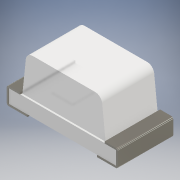
# Autodesk Inventor part: 63-0001
Saved by Autodesk Inventor 2018 (Build 220112000, 112)
## iProperties
Created: 2019-09-26
Part Number: 63-0001
Material: ABS Plastic
Document SubType Name: Modeling
Designer: Bradley
Density: 1.06 g/cm^3
Appearance: Smooth - White
Author: Bradley
Autodesk Inventor part; units mm, degrees
ref_plane "YZ Plane" through (0, 0, 0) normal (1, 0, 0) x (0, 1, 0)
ref_plane "XZ Plane" through (0, 0, 0) normal (0, 1, 0) x (-1, 0, 0)
ref_plane "XY Plane" through (0, 0, 0) normal (0, 0, 1) x (1, 0, 0)
sketch "Sketch1" plane through (0, 0, 0) normal (0, 0, 1) x (1, 0, 0)
  line L0 (-0.775, -0.395) -> (0.775, -0.395)
  line L1 (0.775, -0.395) -> (0.775, 0.395)
  line L2 (0.775, 0.395) -> (-0.775, 0.395)
  line L3 (-0.775, 0.395) -> (-0.775, -0.395)
  line L4 (-0.775, -0.395) -> (0.775, 0.395) construction
  line L5 (0.775, -0.395) -> (-0.775, 0.395) construction
  point P0 (0, 0)
  dimension "d0" = 1.55
  dimension "d1" = 0.79
  constraints: 12 end point, 2 midpoint, 2 parallel, 1 horizontal, 1 perpendicular
  measures "d0" distance of L2.end L1.end
  measures "d1" distance of L1.end L0.end
extrude "Extrusion1" add sketch "Sketch1" along normal blind 0.2
sketch "Sketch2" plane through (0, 0, 0) normal (0, 1, 0) x (-1, 0, 0)
  line L0 (0.775, 0) -> (-0.775, 0) projected
  line L1 (-0.775, 0) -> (-0.775, 0.2) projected
  line L2 (0.775, 0.2) -> (-0.775, 0.2) projected
  line L3 (0.775, 0) -> (0.775, 0.2) projected
  line L4 (0.6, 0.2) -> (0.55, 0.6608)
  arc A0 (0.55, 0.6608) -> (0.4506, 0.75) centre (0.4506, 0.65) ccw
  line L5 (0.4506, 0.75) -> (-0.4506, 0.75)
  arc A1 (-0.4506, 0.75) -> (-0.55, 0.6608) centre (-0.4506, 0.65) ccw
  line L6 (-0.55, 0.6608) -> (-0.6, 0.2)
  line L7 (0.5995, 0.205) -> (-0.5995, 0.205)
  point P0 (0, 0)
  point P1 (0, 0.75)
  point P2 (0, 0.2)
  dimension "d7" = 1.2
  dimension "d8" = 1.1
  dimension "d9" = 0.1
  dimension "d22" = 0.75
  dimension "d23" = 0.005
  constraints: 8 end point, 4 point on circle, 4 point on line, 4 tangent, 2 centre point, 2 horizontal, 2 midpoint, 1 equal length, 1 equal radius, 1 vertical alignment
  measures "d7" distance of L6.end L4.start
  measures "d8" distance of L6.start L4.end
  measures "d9" radius of A0
  measures "d22" distance between parallel lines of L0 L5
  measures "d23" distance between parallel lines of L2 L7
extrude "Extrusion3" add sketch "Sketch2" along normal mid plane 0.75 contours L7 L6 A1 L5 A0 L4
sketch "Sketch3" plane through (-0.775, 0, 0) normal (0, -1, 0) x (1, 0, 0)
  line L0 (0, 0) -> (1.55, 0) projected
  line L1 (1.55, 0) -> (1.55, 0.2) projected
  line L2 (0, 0.2) -> (1.55, 0.2) projected
  line L3 (0, 0) -> (0, 0.2) projected
  line L4 (0, 0.2) -> (1.55, 0.2) projected
  line L5 (0.165, 0.2) -> (0.165, 0.225)
  line L6 (0.165, 0.225) -> (0, 0.225)
  arc A0 (0, 0.225) -> (-0.025, 0.2) centre (0, 0.2) ccw
  line L7 (-0.025, 0.2) -> (-0.025, 0)
  arc A1 (-0.025, 0) -> (0, -0.025) centre (0, 0) ccw
  line L8 (0, -0.025) -> (0.275, -0.025)
  line L9 (0.275, -0.025) -> (0.275, 0)
  line L10 (0, 0) -> (1.55, 0) projected
  line L11 (1.275, 0) -> (1.275, -0.025)
  line L12 (1.275, -0.025) -> (1.55, -0.025)
  arc A2 (1.55, -0.025) -> (1.575, 0) centre (1.55, 0) ccw
  line L13 (1.575, 0) -> (1.575, 0.2)
  arc A3 (1.575, 0.2) -> (1.55, 0.225) centre (1.55, 0.2) ccw
  line L14 (1.55, 0.225) -> (1.385, 0.225)
  line L15 (1.385, 0.225) -> (1.385, 0.2)
  point P0 (0.775, 0)
  dimension "d13" = 1.6
  dimension "d14" = 0.3
  dimension "d15" = 0.19
  constraints: 20 end point, 8 point on circle, 8 point on line, 7 perpendicular, 7 tangent, 4 centre point, 4 coincident, 2 collinear, 1 vertical
  measures "d13" distance between parallel lines of L13 L7
  measures "d14" distance between parallel lines of L7 L9
  measures "d15" distance between parallel lines of L7 L5
extrude "Extrusion4" add sketch "Sketch3" along normal mid plane 0.8 contours L0 L9 L8 A1 L7 A0 L6 L5 L2 L3 | L0 L1 L2 L15 L14 A3 L13 A2 L12 L11
sketch "Sketch4" plane through (0, 0, 0.2) normal (0, 0, 1) x (1, 0, 0)
  line L0 (-0.775, 0.4) -> (-0.775, -0.4) projected
  line L1 (-0.61, -0.4) -> (-0.775, -0.4) projected
  line L2 (-0.61, 0.4) -> (-0.61, -0.4) projected
  line L3 (-0.775, 0.4) -> (-0.61, 0.4) projected
  line L4 (0.61, 0.4) -> (0.61, -0.4) projected
  line L5 (0.775, -0.4) -> (0.61, -0.4) projected
  line L6 (0.775, 0.4) -> (0.775, -0.4) projected
  line L7 (0.61, 0.4) -> (0.775, 0.4) projected
  line L8 (-0.4, -0.15) -> (-0.1, -0.15)
  line L9 (-0.1, -0.15) -> (-0.1, 0.15)
  line L10 (-0.1, 0.15) -> (-0.4, 0.15)
  line L11 (-0.4, 0.15) -> (-0.4, -0.15)
  line L12 (-0.4, -0.15) -> (-0.1, 0.15) construction
  line L13 (-0.1, -0.15) -> (-0.4, 0.15) construction
  point P0 (0, 0)
  point P1 (-0.25, 0)
  point P2 (-0.25, 0)
  dimension "d18" = 0.25
  dimension "d19" = 0.3
  constraints: 12 end point, 3 midpoint, 2 parallel, 2 perpendicular, 1 horizontal, 1 horizontal alignment
  measures "d18" distance of point (0, 0) point (-0.25, 0)
  measures "d19" distance of L9.end L10.end
extrude "Extrusion5" add sketch "Sketch4" along normal blind 0.004 contours L11 L10 L9 L8
body "Solid1"
